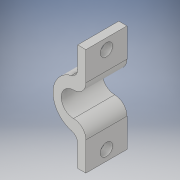
# Autodesk Inventor part: Draht_Halterung
Saved by Autodesk Inventor 2018 (Build 220112000, 112)
## iProperties
Created: 2018-03-14
Part Number: Draht_Halterung
Material: Generisch
Document SubType Name: Modeling
Designer: Julian
Density: 1 g/cm^3
Appearance: Vorgabe
Author: Julian
Autodesk Inventor part; units mm, degrees
ref_plane "YZ Plane" through (0, 0, 0) normal (1, 0, 0) x (0, 1, 0)
ref_plane "XZ Plane" through (0, 0, 0) normal (0, 1, 0) x (-1, 0, 0)
ref_plane "XY Plane" through (0, 0, 0) normal (0, 0, 1) x (1, 0, 0)
sketch "Skizze1" plane through (0, 0, 0) normal (0, 1, 0) x (-1, 0, 0)
  line L0 (0, 0) -> (0, -6)
  line L1 (0, -20) -> (0, -26)
  line L2 (0, -26) -> (2, -26)
  line L3 (2, -26) -> (2, -20.746)
  line L4 (0, 0) -> (2, 0)
  line L5 (2, 0) -> (2, -5.254)
  arc A0 (3, -16) -> (3, -10) centre (3, -13) ccw
  line L6 (6, -13) -> (8, -13)
  line L7 (2, -26) -> (2, -19)
  arc A1 (3.5, -18.8095) -> (3.5, -7.1905) centre (2, -13) ccw
  arc A2 (3.5, -18.8095) -> (2, -20.746) centre (4, -20.746) ccw
  arc A3 (2, -5.254) -> (3.5, -7.1905) centre (4, -5.254) ccw
  line L8 (3, -16) -> (3, -16)
  line L9 (0, -19) -> (0, -20)
  line L10 (3, -10) -> (3, -10)
  line L11 (0, -7) -> (0, -6)
  arc A4 (3, -16) -> (0, -19) centre (3, -19) ccw
  arc A5 (0, -7) -> (3, -10) centre (3, -7) ccw
  point P0 (0, -10)
  point P1 (0, -16)
  point P2 (2, -19)
  point P3 (2, -7)
  dimension "d0" = 10
  dimension "d1" = 3
  dimension "d3" = 10
  dimension "d4" = 2
  dimension "d5" = 7
  dimension "d6" = 2
  dimension "d7" = 7
  dimension "d9" = 3
  dimension "d23" = 2
  dimension "d24" = 7
  dimension "d25" = 2
  dimension "d26" = 3
  constraints: 24 end point, 16 point on circle, 10 point on line, 8 tangent, 6 centre point, 6 perpendicular, 3 horizontal, 2 equal radius, 2 vertical
  measures "d0" distance of L0.start point (0, -10)
  measures "d1" distance of point (0, -10) L10.start
  measures "d3" distance of point (0, -16) L1.end
  measures "d4" distance of L1.end L2.end
  measures "d5" distance of L2.end point (2, -19)
  measures "d6" distance of L0.start L4.end
  measures "d7" distance of L4.end point (2, -7)
  measures "d9" radius of A0
  measures "d23" distance of L6.start L6.end
  measures "d24" distance of L2.end L7.end
  measures "d25" radius of A2
  measures "d26" radius of A4
extrude "Extrusion1" add sketch "Skizze1" along normal blind 10
sketch "Skizze2" plane through (-2, 0, -5) normal (-1, 0, 0) x (0, 0, 1)
  line L0 (5, 0) -> (5, 10) projected
  line L1 (5, 5) -> (2.5, 5)
  line L2 (-21, 0) -> (-21, 10) projected
  line L3 (-21, 5) -> (-18.5, 5)
  dimension "d14" = 2.5
  dimension "d15" = 2.5
  constraints: 4 end point, 2 horizontal, 2 midpoint
  measures "d14" distance of L1.start L1.end
  measures "d15" distance of L3.start L3.end
hole "Bohrung1" at (-2, 5, -2.5) at (-2, 5, -23.5) direction (1, 0, 0) diameter 3 depth 8 tip angle 118
